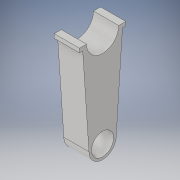
# Autodesk Inventor part: PistonsRod
Saved by Autodesk Inventor 2018 (Build 220112000, 112)
## iProperties
Created: 2019-09-03
Part Number: PistonsRod
Material: Generic
Document SubType Name: Modeling
Designer: 871357
Density: 1 g/cm^3
Appearance: Default
Author: 871357
Autodesk Inventor part; units mm, degrees
ref_plane "YZ Plane" through (0, 0, 0) normal (1, 0, 0) x (0, 1, 0)
sketch "Sketch1" plane through (0, 0, 0) normal (0, 1, 0) x (-1, 0, 0)
  circle A0 centre (0, 0) radius 43.18
  dimension "d0" = 86.36
  constraints: 1 centre point, 1 coincident
  measures "d0" diameter of A0
extrude "Extrusion1" add sketch "Sketch1" against normal blind 63.5
sketch "Sketch2" plane through (0, 0, 0) normal (0, 0, 1) x (1, 0, 0)
  line L0 (-43.18, 0) -> (43.18, 0) projected
  arc A0 (-43.18, 0) -> (43.18, 0) centre (0, 24.003) ccw
  line L1 (-43.18, -63.5) -> (43.18, -63.5) projected
  point P0 (0, 0)
  dimension "d4" = 38.1
  constraints: 2 point on circle, 1 centre point
  measures "d4" distance edge to line of A0 L1
extrude "Extrusion2" cut sketch "Sketch2" along normal mid plane 101.6
ref_plane "Work Plane1" through (0, 0, 0) normal (0, -1, 0) x (1, 0, 0)
sketch "Sketch3" plane through (0, 0, 0) normal (0, -1, 0) x (1, 0, 0)
  circle A0 centre (0, 0) radius 38.1
  dimension "d8" = 76.2
  constraints: 1 centre point, 1 coincident
  measures "d8" diameter of A0
extrude "Extrusion3" cut sketch "Sketch3" along normal blind 57.15
sketch "Sketch4" plane through (0, 0, 0) normal (1, 0, 0) x (0, 1, 0)
  circle A0 centre (-25.4, 0) radius 12.7
  point P0 (0, 0)
  dimension "d11" = 25.4
  dimension "d12" = 25.4
  dimension "d13" = 0
  constraints: 1 centre point
  measures "d11" diameter of A0
  measures "d12" distance of A0.centre point (0, 0)
  measures "d13" vertical distance of point (0, 0) A0.centre
extrude "Extrusion4" add sketch "Sketch4" along normal mid plane 78.74
sketch "Sketch5" plane through (0, 0, 0) normal (1, 0, 0) x (0, 1, 0)
  circle A0 centre (-25.4, 0) radius 13.97
  arc A1 (-25.4, 17.145) -> (-25.4, -17.145) centre (-25.4, 0) ccw
  line L0 (-63.5, 43.18) -> (-63.5, -43.18) projected
  circle A2 centre (93.98, 0) radius 20.32
  arc A3 (90.484, -25.1583) -> (93.98, 25.4) centre (93.98, 0) ccw
  line L1 (93.98, 25.4) -> (-25.4, 17.145)
  line L2 (90.484, -25.1583) -> (-25.4, -17.145)
  point P0 (0, 0)
  point P1 (-25.4, 12.7)
  dimension "d16" = 27.94
  dimension "d17" = 34.29
  dimension "d18" = 38.1
  dimension "d19" = 43.18
  dimension "d20" = 40.64
  dimension "d21" = 0
  dimension "d22" = 119.38
  dimension "d23" = 50.8
  constraints: 4 centre point, 4 end point, 4 point on circle, 2 coincident
  measures "d16" diameter of A0
  measures "d17" diameter of A1
  measures "d18" distance from line of L0 A0.centre
  measures "d19" vertical distance of L0.start A0.centre
  measures "d20" diameter of A2
  measures "d21" vertical distance of A0.centre A2.centre
  measures "d22" distance of A0.centre A2.centre
  measures "d23" diameter of A3
extrude "Extrusion5" add sketch "Sketch5" along normal mid plane 31.75
sketch "Sketch6" plane through (0, 0, 0) normal (1, 0, 0) x (0, 1, 0)
  circle A0 centre (93.98, 0) radius 20.32 construction
  line L0 (93.98, 0) -> (93.98, -43.5701)
  line L1 (93.98, 0) -> (93.98, 40.9183)
  line L2 (93.98, 40.9183) -> (142.8926, 40.9183)
  line L3 (142.8926, 40.9183) -> (133.2711, -47.8298)
  line L4 (133.2711, -47.8298) -> (93.98, -43.5701)
  point P0 (0, 0)
  constraints: 10 end point, 2 perpendicular, 2 vertical
extrude "Extrusion6" cut sketch "Sketch6" along normal mid plane 2540
ref_plane "Work Plane2" through (0, 0, -22.86) normal (0, 0, 1) x (1, 0, 0)
sketch "Sketch7" plane through (0, 0, -22.86) normal (0, 0, 1) x (1, 0, 0)
  line L0 (15.875, 90.484) -> (15.875, 93.98) projected
  line L1 (-15.875, -25.4) -> (-15.875, 93.98) construction
  line L2 (15.875, 93.98) -> (-15.875, 93.98)
  line L3 (-15.875, 93.98) -> (-15.875, 88.9)
  line L4 (-15.875, 88.9) -> (15.875, 88.9)
  line L5 (15.875, 88.9) -> (15.875, 93.98)
  point P0 (0, 0)
  dimension "d29" = 5.08
  constraints: 8 end point, 2 parallel, 1 horizontal, 1 perpendicular, 1 point on line
  measures "d29" distance of L4.end L0.end
extrude "Extrusion7" add sketch "Sketch7" against normal blind 6.35
mirror "Mirror1" about plane through (0, 0, 0) normal (0, 0, 1) of "Extrusion7"
sketch "Sketch8" plane through (15.875, 0, 0) normal (1, 0, 0) x (0, 0, -1)
  circle A0 centre (0, -25.4) radius 13.97 projected
  line L0 (-20.32, 93.98) -> (-29.21, 93.98) projected
  arc A1 (-20.32, 93.98) -> (20.32, 93.98) centre (0, 93.98) ccw projected
  line L1 (20.32, 93.98) -> (29.21, 93.98) projected
  line L2 (29.21, 88.9) -> (29.21, 93.98) projected
  line L3 (25.0487, 88.9) -> (29.21, 88.9) projected
  line L4 (25.0487, 88.9) -> (17.145, -25.4) projected
  arc A2 (-17.145, -25.4) -> (17.145, -25.4) centre (0, -25.4) ccw projected
  line L5 (-17.145, -25.4) -> (-25.0487, 88.9) projected
  line L6 (-25.0487, 88.9) -> (-29.21, 88.9) projected
  line L7 (-29.21, 88.9) -> (-29.21, 93.98) projected
  point P0 (0, 0)
extrude "Extrusion8" cut sketch "Sketch8" against normal blind 38.1 keep common part
body "Solid1"
